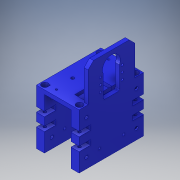
# Autodesk Inventor part: КВ33.044.501 - Каретка оси Y
Saved by Autodesk Inventor 2019 (Build 230136000, 136)
## iProperties
Created: 2019-07-21
Part Number: КВ33.044.501 - Каретка оси Y
Material: Пластик АБС
Document SubType Name: Modeling
Designer: Петров Иван
Density: 1.06 g/cm^3
Appearance: Синий — малярная краска — глянцевая
Mass: 139.056 g
Surface Area: 506.094 cm^2
Volume: 131.185 cm^3
Author: Петров Иван
Autodesk Inventor part; units mm, degrees
(part 1 of 2)
ref_plane "YZ Plane" through (0, 0, 0) normal (1, 0, 0) x (0, 1, 0)
ref_plane "XZ Plane" through (0, 0, 0) normal (0, 1, 0) x (-1, 0, 0)
ref_plane "XY Plane" through (0, 0, 0) normal (0, 0, 1) x (1, 0, 0)
sketch "Эскиз1" plane through (0, 0, 0) normal (1, 0, 0) x (0, 1, 0)
  line L0 (-34, 40) -> (34, 40)
  line L1 (34, 40) -> (34, -40)
  line L2 (34, -40) -> (-34, -40)
  line L3 (-34, -40) -> (-34, 40)
  line L4 (-34, 40) -> (34, -40) construction
  line L5 (34, 40) -> (-34, -40) construction
  line L6 (0, 0) -> (0, 31)
  line L7 (0, 31) -> (21.3, 31)
  line L8 (0, 31) -> (-21.3, 31)
  line L9 (0, 0) -> (0, -31)
  line L10 (0, -31) -> (21.3, -31)
  line L11 (0, -31) -> (-21.3, -31)
  circle A0 centre (21.3, 31) radius 2.1
  circle A1 centre (-21.3, 31) radius 2.1
  circle A2 centre (21.3, -31) radius 2.1
  circle A3 centre (-21.3, -31) radius 2.1
  dimension "d0" = 68
  dimension "d1" = 80
  dimension "d2" = 21.3
  dimension "d3" = 21.3
  dimension "d4" = 31
  dimension "d5" = 31
  dimension "d6" = 21.3
  dimension "d7" = 21.3
  dimension "d8" = 4.2
  dimension "d9" = 4.2
  dimension "d10" = 4.2
  dimension "d11" = 4.2
  constraints: 24 end point, 4 centre point, 4 coincident, 3 horizontal, 3 perpendicular, 2 midpoint, 2 parallel, 2 vertical
  measures "d0" distance of L1.end L2.end
  measures "d1" distance of L0.end L1.end
  measures "d2" distance of L6.end L7.end
  measures "d3" distance of L6.end L8.end
  measures "d4" distance of L6.start L6.end
  measures "d5" distance of L6.start L9.end
  measures "d6" distance of L9.end L10.end
  measures "d7" distance of L9.end L11.end
  measures "d8" diameter of A0
  measures "d9" diameter of A1
  measures "d10" diameter of A2
  measures "d11" diameter of A3
extrude "Выдавливание1" add sketch "Эскиз1" along normal blind 10
sketch "Эскиз2" plane through (10, 0, 0) normal (1, 0, 0) x (0, 0, -1)
  line L0 (-40, 34) -> (-40, -34) projected
  line L1 (-40, 0) -> (-40, 5)
  line L2 (-40, 0) -> (-26, 0)
  line L3 (-26, 0) -> (-26, 11)
  line L4 (-40, 5) -> (-26, 5)
  line L5 (-26, 5) -> (-26, 11)
  line L6 (-26, 11) -> (-40, 11)
  line L7 (-40, 11) -> (-40, 5)
  line L8 (-40, 0) -> (-40, -5)
  line L9 (-26, 0) -> (-26, -11)
  line L10 (-40, -5) -> (-26, -5)
  line L11 (-26, -5) -> (-26, -11)
  line L12 (-26, -11) -> (-40, -11)
  line L13 (-40, -11) -> (-40, -5)
  line L14 (40, -34) -> (40, 34) projected
  line L15 (40, 0) -> (40, 5)
  line L16 (40, 0) -> (26, 0)
  line L17 (26, 0) -> (26, 11)
  line L18 (26, 11) -> (40, 11)
  line L19 (40, 11) -> (40, 5)
  line L20 (40, 5) -> (26, 5)
  line L21 (26, 5) -> (26, 11)
  line L22 (26, 0) -> (26, -11)
  line L23 (40, 0) -> (40, -5)
  line L24 (26, -11) -> (40, -11)
  line L25 (40, -11) -> (40, -5)
  line L26 (40, -5) -> (26, -5)
  line L27 (26, -5) -> (26, -11)
  point P0 (0, 0)
  dimension "d14" = 5
  dimension "d15" = 14
  dimension "d16" = 11
  dimension "d17" = 5
  dimension "d18" = 11
  dimension "d19" = 5
  dimension "d20" = 14
  dimension "d21" = 11
  dimension "d22" = 11
  dimension "d23" = 5
  constraints: 52 end point, 8 parallel, 7 perpendicular, 5 horizontal, 4 point on line, 2 midpoint, 2 vertical
  measures "d14" distance of L1.start L1.end
  measures "d15" distance of L1.start L2.end
  measures "d16" distance of L2.end L3.end
  measures "d17" distance of L1.start L8.end
  measures "d18" distance of L2.end L9.end
  measures "d19" distance of L15.start L15.end
  measures "d20" distance of L15.start L16.end
  measures "d21" distance of L16.end L17.end
  measures "d22" distance of L16.end L22.end
  measures "d23" distance of L15.start L23.end
extrude "Выдавливание2" cut sketch "Эскиз2" against normal blind 10 contours L6 L3 L4 L0 | L10 L9 L12 L0 | L24 L22 L26 L14 | L20 L17 L18 L14
sketch "Эскиз3" plane through (0, 34, 40) normal (0, 1, 0) x (1, 0, 0)
  line L0 (0, 0) -> (10, 0) projected
  line L1 (5, 0) -> (5, 11.1)
  line L2 (0, 11.1) -> (10, 11.1) projected
  circle A0 centre (5, 5.55) radius 1.8
  line L3 (0, 80) -> (10, 80) projected
  line L4 (5, 80) -> (5, 68.9)
  line L5 (0, 68.9) -> (10, 68.9) projected
  circle A1 centre (5, 74.45) radius 1.8
  point P0 (0, 40)
  dimension "d26" = 3.6
  dimension "d29" = 3.6
  constraints: 6 midpoint, 4 end point, 2 centre point
  measures "d26" diameter of A0
  measures "d29" diameter of A1
extrude "Выдавливание3" cut sketch "Эскиз3" against normal through all
sketch "Эскиз4" plane through (0, 34, 40) normal (0, 1, 0) x (1, 0, 0)
  circle A0 centre (5, 5.55) radius 1.8 projected
  circle A1 centre (5, 5.55) radius 4
  circle A2 centre (5, 74.45) radius 1.8 projected
  circle A3 centre (5, 74.45) radius 4
  point P0 (0, 40)
  dimension "d30" = 8
  dimension "d31" = 8
  constraints: 2 centre point, 2 coincident
  measures "d30" diameter of A1
  measures "d31" diameter of A3
extrude "Выдавливание4" cut sketch "Эскиз4" against normal blind 10
sketch "Эскиз5" plane through (10, 0, 0) normal (1, 0, 0) x (0, 0, -1)
  line L0 (0, 0) -> (0, 18)
  line L1 (0, 18) -> (0, 20)
  line L2 (0, 20) -> (-15, 20)
  line L3 (-15, 20) -> (15, 20)
  circle A0 centre (-15, 20) radius 1.5
  circle A1 centre (15, 20) radius 1.5
  line L4 (0, 0) -> (6.6954, 0)
  line L5 (0, -18) -> (0, -20)
  line L6 (0, -20) -> (-15, -20)
  line L7 (-15, -20) -> (15, -20)
  circle A2 centre (-15, -20) radius 1.5
  circle A3 centre (15, -20) radius 1.5
  dimension "d34" = 18
  dimension "d35" = 2
  dimension "d36" = 15
  dimension "d37" = 30
  dimension "d38" = 3
  dimension "d39" = 3
  constraints: 16 end point, 6 symmetric about line, 4 centre point, 4 coincident, 3 point on line, 2 horizontal, 1 vertical, 2 other
  measures "d34" distance of L0.start L0.end
  measures "d35" distance of L0.end L1.end
  measures "d36" distance of L1.end L2.end
  measures "d37" distance of L2.end L3.end
  measures "d38" diameter of A0
  measures "d39" diameter of A1
extrude "Выдавливание5" cut sketch "Эскиз5" against normal blind 10 contours A2 | A3
sketch "Эскиз6" plane through (10, 0, 0) normal (1, 0, 0) x (0, 0, -1)
  circle A0 centre (15, -20) radius 1.5 projected
  circle A1 centre (-15, -20) radius 1.5 projected
  circle A2 centre (-31, 21.3) radius 2.1 projected
  circle A3 centre (-31, -21.3) radius 2.1 projected
  circle A4 centre (31, 21.3) radius 2.1 projected
  circle A5 centre (31, -21.3) radius 2.1 projected
  line L0 (-40, 11) -> (-26, 11) projected
  line L1 (-26, 11) -> (-26, 5) projected
  line L2 (-26, 5) -> (-40, 5) projected
  line L3 (-40, 5) -> (-40, -5) projected
  line L4 (-40, -5) -> (-26, -5) projected
  line L5 (-26, -5) -> (-26, -11) projected
  line L6 (-26, -11) -> (-40, -11) projected
  line L7 (-40, -11) -> (-40, -34) projected
  line L8 (-40, -34) -> (40, -34) projected
  line L9 (40, -34) -> (40, -11) projected
  line L10 (40, -11) -> (26, -11) projected
  line L11 (26, -11) -> (26, -5) projected
  line L12 (26, -5) -> (40, -5) projected
  line L13 (40, -5) -> (40, 5) projected
  line L14 (40, 5) -> (26, 5) projected
  line L15 (26, 5) -> (26, 11) projected
  line L16 (26, 11) -> (40, 11) projected
  line L17 (40, 11) -> (40, 34) projected
  line L18 (40, 34) -> (-40, 34) projected
  line L19 (-40, 34) -> (-40, 11) projected
  point P0 (0, 0)
sketch "Эскиз8" plane through (0, 0, 0) normal (-1, 0, 0) x (0, 0, 1)
  line L0 (-40, 34) -> (-40, 11) projected
  line L1 (40, 11) -> (40, 34) projected
  line L2 (-40, 34) -> (40, 34)
  line L3 (40, 34) -> (40, 29)
  line L4 (40, 29) -> (-40, 29)
  line L5 (-40, 29) -> (-40, 34)
  point P0 (0, 0)
  dimension "d46" = 5
  constraints: 8 end point, 2 parallel, 1 horizontal, 1 perpendicular, 1 point on line
  measures "d46" distance of L2.end L3.end
extrude "Выдавливание7" add sketch "Эскиз8" along normal blind 33
sketch "Эскиз13" plane through (-33, 0, 0) normal (-1, 0, 0) x (0, 0, 1)
  circle A0 centre (15, -20) radius 1.5
  circle A1 centre (-15, -20) radius 1.5
  circle A2 centre (-31, 21.3) radius 2.1
  circle A3 centre (-31, -21.3) radius 2.1
  circle A4 centre (31, 21.3) radius 2.1
  circle A5 centre (31, -21.3) radius 2.1
  line L0 (-40, 11) -> (-26, 11)
  line L1 (-26, 11) -> (-26, 5)
  line L2 (-26, 5) -> (-40, 5)
  line L3 (-40, 5) -> (-40, -5)
  line L4 (-40, -5) -> (-26, -5)
  line L5 (-26, -5) -> (-26, -11)
  line L6 (-26, -11) -> (-40, -11)
  line L7 (-40, -11) -> (-40, -34)
  line L8 (-40, -34) -> (40, -34)
  line L9 (40, -34) -> (40, -11)
  line L10 (40, -11) -> (26, -11)
  line L11 (26, -11) -> (26, -5)
  line L12 (26, -5) -> (40, -5)
  line L13 (40, -5) -> (40, 5)
  line L14 (40, 5) -> (26, 5)
  line L15 (26, 5) -> (26, 11)
  line L16 (26, 11) -> (40, 11)
  line L17 (40, 11) -> (40, 34)
  line L18 (40, 34) -> (-40, 34)
  line L19 (-40, 34) -> (-40, 11)
  point P0 (0, 0)
  point P1 (0, 0)
  constraints: 40 end point, 6 centre point
extrude "Выдавливание11" add sketch "Эскиз13" along normal blind 10
sketch "Эскиз14" plane through (10, 34, 40) normal (0, 1, 0) x (1, 0, 0)
  line L0 (0, 80) -> (-53, 80) projected
  line L1 (-26.5, 80) -> (-26.5, 69.4857)
  circle A0 centre (-5, 5.55) radius 4 projected
  circle A1 centre (-5, 74.45) radius 4 projected
  line L2 (0, 0) -> (-53, 0) projected
  line L3 (0, 80) -> (0, 0) projected
  line L4 (0, 80) -> (-53, 80) projected
  line L5 (-53, 0) -> (-53, 80) projected
  circle A2 centre (-5, 5.55) radius 1.8 projected
  circle A3 centre (-5, 74.45) radius 1.8 projected
  circle A4 centre (-48, 5.55) radius 1.8
  circle A5 centre (-48, 74.45) radius 1.8
  point P0 (-10, 40)
  constraints: 2 centre point, 2 end point, 2 symmetric about line, 1 midpoint, 1 vertical, 2 other
extrude "Выдавливание12" cut sketch "Эскиз14" against normal through all contours A4 | A5
sketch "Эскиз15" plane through (10, 34, 40) normal (0, 1, 0) x (1, 0, 0)
  circle A0 centre (-48, 74.45) radius 1.8 projected
  circle A1 centre (-48, 74.45) radius 4
  circle A2 centre (-48, 5.55) radius 1.8 projected
  circle A3 centre (-48, 5.55) radius 4
  point P0 (-10, 40)
  dimension "d65" = 8
  dimension "d66" = 8
  constraints: 2 centre point, 2 coincident
  measures "d65" diameter of A1
  measures "d66" diameter of A3
extrude "Выдавливание13" cut sketch "Эскиз15" against normal blind 20
sketch "Эскиз16" plane through (10, 34, 40) normal (0, 1, 0) x (1, 0, 0)
  circle A0 centre (-48, 74.45) radius 4 projected
  circle A1 centre (-48, 5.55) radius 4 projected
  circle A2 centre (-5, 5.55) radius 4 projected
  circle A3 centre (-5, 74.45) radius 4 projected
  line L0 (0, 0) -> (-53, 0) projected
  line L1 (0, 80) -> (0, 0) projected
  line L2 (0, 80) -> (-53, 80) projected
  line L3 (-53, 0) -> (-53, 80) projected
  point P0 (-10, 40)
sketch "Эскиз17" plane through (-33, -34, -40) normal (0, -1, 0) x (1, 0, 0)
  circle A0 centre (-5, 5.55) radius 4
  circle A1 centre (-5, 74.45) radius 4
  circle A2 centre (-5, 5.55) radius 1.8 projected
  line L0 (-5, 5.55) -> (-5, 18.1127)
  circle A3 centre (38, 74.45) radius 4
  circle A4 centre (38, 5.55) radius 4
  circle A5 centre (-5, 5.55) radius 4
  circle A6 centre (-5, 74.45) radius 4
  line L1 (-10, 0) -> (43, 0)
  line L2 (-10, 80) -> (-10, 0)
  line L3 (-10, 80) -> (43, 80)
  line L4 (43, 0) -> (43, 80)
  circle A7 centre (-5, 5.55) radius 1.8
  point P0 (33, 40)
  point P1 (-10, 40)
  point P2 (0, 40)
  constraints: 10 end point, 7 centre point, 1 symmetric about line, 1 vertical, 3 other
extrude "Выдавливание14" cut sketch "Эскиз17" against normal blind 20 contours A0 | A1 | A3 | A4
sketch "Эскиз25" plane through (10, 34, 40) normal (0, 1, 0) x (1, 0, 0)
  line L0 (-10, 68.9) -> (0, 68.9) projected
  line L1 (-10, 11.1) -> (0, 11.1) projected
  line L2 (-5, 68.9) -> (0, 68.9)
  line L3 (0, 68.9) -> (0, 11.1)
  line L4 (0, 11.1) -> (-5, 11.1)
  line L5 (-5, 11.1) -> (-5, 68.9)
  point P0 (-10, 40)
  constraints: 8 end point, 2 parallel, 1 horizontal, 1 midpoint, 1 perpendicular, 1 point on line
extrude "Выдавливание21" add sketch "Эскиз25" along normal blind 40
sketch "Эскиз26" plane through (10, 0, 0) normal (1, 0, 0) x (0, 0, -1)
  line L0 (-12.6, 44.2) -> (-14.9, 44.2)
  line L1 (-12.6, 44.2) -> (-12.6, 42.8)
  line L2 (-14.9, 42.8) -> (-12.6, 42.8)
  line L3 (-14.9, 36.2) -> (-14.9, 42.8)
  line L4 (-12.6, 36.2) -> (-14.9, 36.2)
  circle A0 centre (0, 62) radius 9.15
  circle A1 centre (0, 62) radius 1.5
  circle A2 centre (8, 26) radius 1.3
  circle A3 centre (13.5, 39.5) radius 1.3
  circle A4 centre (13.5, 31.5) radius 1.3
  circle A5 centre (13.5, 47.5) radius 1.3
  circle A6 centre (13.5, 55.5) radius 1.3
  circle A7 centre (-8, 26) radius 1.3
  circle A8 centre (-13.5, 39.5) radius 1.3
  circle A9 centre (-13.5, 31.5) radius 1.3
  circle A10 centre (-13.5, 47.5) radius 1.3
  circle A11 centre (-13.5, 55.5) radius 1.3
  line L5 (-0.1, 73.0198) -> (-0.1, 72.4796)
  line L6 (-7, 73.0198) -> (-0.1, 73.0198)
  arc A12 (-7, 73.0198) -> (-7.75, 72.9686) centre (-7, 67.5) ccw
  line L7 (-7.75, 70.5) -> (-7.75, 72.9686)
  arc A13 (-9.5, 68.75) -> (-7.75, 70.5) centre (-9.5, 70.5) ccw
  line L8 (-10, 68.75) -> (-9.5, 68.75)
  line L9 (-10, 31.1937) -> (-10, 68.75)
  arc A14 (-10, 31.1937) -> (-9.6078, 30.5055) centre (-9.2, 31.1937) ccw
  arc A15 (-9.6078, 30.5055) -> (-8.9945, 29.8922) centre (-10.5, 29) ccw
  arc A16 (-8.9945, 29.8922) -> (-8.3063, 29.5) centre (-8.3063, 30.3) ccw
  line L10 (8.3063, 29.5) -> (-8.3063, 29.5)
  arc A17 (8.3063, 29.5) -> (8.9945, 29.8922) centre (8.3063, 30.3) ccw
  arc A18 (9.6078, 30.5055) -> (8.9945, 29.8922) centre (10.5, 29) ccw
  arc A19 (8.9945, 29.8922) -> (9.6078, 30.5055) centre (10.5, 29) ccw
  line L11 (-11.3229, 68.75) -> (-10, 68.75)
  arc A20 (-11.3229, 68.75) -> (-11.5, 67.4989) centre (-6.9922, 67.4989) ccw
  line L12 (-11.5, 67.4989) -> (-11.5, 60)
  line L13 (-12.6, 60) -> (-11.5, 60)
  line L14 (-12.6, 58.8) -> (-12.6, 60)
  line L15 (-14.9, 58.8) -> (-12.6, 58.8)
  line L16 (-14.9, 52.2) -> (-14.9, 58.8)
  line L17 (-12.6, 52.2) -> (-14.9, 52.2)
  line L18 (-12.6, 50.8) -> (-12.6, 52.2)
  line L19 (-14.9, 50.8) -> (-12.6, 50.8)
  line L20 (-14.9, 44.2) -> (-14.9, 50.8)
  line L21 (-12.6, 44.2) -> (-14.9, 44.2)
  line L22 (-12.6, 42.8) -> (-12.6, 44.2)
  line L23 (-14.9, 42.8) -> (-12.6, 42.8)
  line L24 (-14.9, 36.2) -> (-14.9, 42.8)
  line L25 (-12.6, 36.2) -> (-14.9, 36.2)
  line L26 (-12.6, 34.8) -> (-12.6, 36.2)
  line L27 (-14.9, 34.8) -> (-12.6, 34.8)
  line L28 (-14.9, 28.2) -> (-14.9, 34.8)
  line L29 (-12.6, 28.2) -> (-14.9, 28.2)
  line L30 (-12.6, 26.9802) -> (-12.6, 28.2)
  arc A21 (-12.6, 26.9802) -> (-12.5198, 26.9) centre (-11.5, 28) ccw
  line L31 (-11.3, 26.9) -> (-12.5198, 26.9)
  line L32 (-11.3, 24.6) -> (-11.3, 26.9)
  line L33 (-4.7, 24.6) -> (-11.3, 24.6)
  line L34 (-4.7, 26.9) -> (-4.7, 24.6)
  line L35 (4.7, 26.9) -> (-4.7, 26.9)
  line L36 (4.7, 24.6) -> (4.7, 26.9)
  line L37 (11.3, 24.6) -> (4.7, 24.6)
  line L38 (11.3, 26.9) -> (11.3, 24.6)
  line L39 (12.5198, 26.9) -> (11.3, 26.9)
  arc A22 (12.5198, 26.9) -> (12.6, 26.9802) centre (11.5, 28) ccw
  line L40 (12.6, 28.2) -> (12.6, 26.9802)
  line L41 (14.9, 28.2) -> (12.6, 28.2)
  line L42 (14.9, 34.8) -> (14.9, 28.2)
  line L43 (12.6, 34.8) -> (14.9, 34.8)
  line L44 (12.6, 36.2) -> (12.6, 34.8)
  line L45 (14.9, 36.2) -> (12.6, 36.2)
  line L46 (14.9, 42.8) -> (14.9, 36.2)
  line L47 (12.6, 42.8) -> (14.9, 42.8)
  line L48 (12.6, 44.2) -> (12.6, 42.8)
  line L49 (14.9, 44.2) -> (12.6, 44.2)
  line L50 (14.9, 50.8) -> (14.9, 44.2)
  line L51 (12.6, 50.8) -> (14.9, 50.8)
  line L52 (12.6, 52.2) -> (12.6, 50.8)
  line L53 (14.9, 52.2) -> (12.6, 52.2)
  line L54 (14.9, 58.8) -> (14.9, 52.2)
  line L55 (12.6, 58.8) -> (14.9, 58.8)
  line L56 (12.6, 60) -> (12.6, 58.8)
  line L57 (11.5, 60) -> (12.6, 60)
  line L58 (11.5, 67.5) -> (11.5, 60)
  arc A23 (11.5, 67.5) -> (11.3229, 68.75) centre (6.9922, 67.4989) ccw
  line L59 (10, 68.75) -> (11.3229, 68.75)
  line L60 (9.5, 68.75) -> (10, 68.75)
  arc A24 (7.75, 70.5) -> (9.5, 68.75) centre (9.5, 70.5) ccw
  line L61 (7.75, 72.9686) -> (7.75, 70.5)
  arc A25 (7.75, 72.9686) -> (7, 73.0198) centre (7, 67.5) ccw
  line L62 (0.1, 73.0198) -> (7, 73.0198)
  line L63 (0.1, 72.4796) -> (0.1, 73.0198)
  arc A26 (-8.9945, 29.8922) -> (-9.6078, 30.5055) centre (-10.5, 29) ccw
  arc A27 (9.6078, 30.5055) -> (10, 31.1895) centre (9.2, 31.1937) ccw
  line L64 (10, 68.75) -> (10, 31.1895)
  line L65 (0, 0) -> (0, 74)
  line L66 (28.9, 74) -> (-28.9, 74) projected
  line L67 (0, 74) -> (0, 62)
  line L68 (-9.15, 62) -> (-10, 62)
  line L69 (9.15, 62) -> (10, 62)
  point P0 (0, 62)
  dimension "d102" = 12
  constraints: 138 end point, 34 point on circle, 28 centre point, 5 point on line, 1 midpoint, 1 perpendicular
  measures "d102" distance of L65.end L67.end
extrude "Выдавливание22" cut sketch "Эскиз26" against normal blind 5 contours L68 A0 L65 L10 A16 A26 A14 L9 | A0 L65 A1 | A0 L65 A1 | A0 L69 L64 A27 A18 A17 L10 L65 | L65 A1 | A1 L65 | A3 | A5 | A6 | A8 | A10 | A11
sketch "Эскиз29" plane through (-43, 34, -40) normal (0, 1, 0) x (1, 0, 0)
  line L0 (43, -11.1) -> (53, -11.1) projected
  line L1 (48, -11.1) -> (48, -68.9) projected
  line L2 (48, -11.1) -> (48, -68.9)
  circle A0 centre (40.9968, -58.9777) radius 1.5
  line L3 (33.923, -34.3302) -> (33.923, -66.4777)
  line L4 (33.923, -66.4777) -> (47.9968, -66.4777)
  line L5 (47.9968, -66.4777) -> (47.9968, -34.3302)
  line L6 (47.9968, -34.3302) -> (33.923, -34.3302)
  point P0 (43, -40)
  point P1 (40.9968, -50.4777)
  constraints: 10 end point, 1 centre point, 1 collinear, 1 midpoint
extrude "Выдавливание23" cut sketch "Эскиз29" against normal blind 4 contours A0 | L6 L5 L4 L3
chamfer "Фаска5" distance 2.75 angle 45 2 edges at (7.5, 74, 28.9) (7.5, 74, -28.9)
sketch "Эскиз43" plane through (-43, 34, 40) normal (0, 1, 0) x (1, 0, 0)
  line L0 (1.9345, -0.1187) -> (2.4471, -0.1187)
  line L1 (2.4471, -0.1187) -> (2.5388, 1.3153)
  arc A0 (6.7302, 1.3153) -> (2.5388, 1.3153) centre (4.6345, 1.1813) ccw
  line L2 (6.7302, 1.3153) -> (6.8219, -0.1187)
  line L3 (6.8219, -0.1187) -> (11.1103, -0.1187)
  arc A1 (11.1103, -0.1187) -> (11.181, -0.0894) centre (11.1103, -0.0187) ccw
  line L4 (11.181, -0.0894) -> (11.5052, 0.2348)
  arc A2 (11.8588, 0.3813) -> (11.5052, 0.2348) centre (11.8588, -0.1187) ccw
  line L5 (11.8588, 0.3813) -> (21.5345, 0.3813)
  arc A3 (21.5345, 0.3813) -> (21.4407, 0.4466) centre (21.5345, 0.4813) ccw
  line L6 (21.4407, 0.4466) -> (21.4407, 9.5417)
  arc A4 (21.4407, 9.5417) -> (21.4519, 9.7313) centre (21.5345, 9.6313) ccw
  line L7 (21.4519, 9.7313) -> (18.6088, 9.7313)
  arc A5 (18.2552, 9.8777) -> (18.6088, 9.7313) centre (18.6088, 10.2313) ccw
  line L8 (18.2552, 9.8777) -> (17.931, 10.202)
  arc A6 (17.931, 10.202) -> (17.8603, 10.2313) centre (17.8603, 10.1313) ccw
  line L9 (17.8603, 10.2313) -> (15.1088, 10.2313)
  arc A7 (15.1088, 10.2313) -> (15.0381, 10.202) centre (15.1088, 10.1313) ccw
  line L10 (15.0381, 10.202) -> (14.7138, 9.8777)
  arc A8 (14.3603, 9.7313) -> (14.7138, 9.8777) centre (14.3603, 10.2313) ccw
  line L11 (14.3603, 9.7313) -> (9.1088, 9.7313)
  arc A9 (8.7552, 9.8777) -> (9.1088, 9.7313) centre (9.1088, 10.2313) ccw
  line L12 (8.7552, 9.8777) -> (8.431, 10.202)
  arc A10 (8.431, 10.202) -> (8.3603, 10.2313) centre (8.3603, 10.1313) ccw
  line L13 (8.3603, 10.2313) -> (5.6088, 10.2313)
  arc A11 (5.6088, 10.2313) -> (5.5381, 10.202) centre (5.6088, 10.1313) ccw
  line L14 (5.5381, 10.202) -> (5.2138, 9.8777)
  arc A12 (4.8603, 9.7313) -> (5.2138, 9.8777) centre (4.8603, 10.2313) ccw
  line L15 (4.8603, 9.7313) -> (1.9345, 9.7313)
  arc A13 (1.9345, 9.7313) -> (2.0046, 9.5599) centre (1.9345, 9.6313) ccw
  line L16 (2.0046, 9.5599) -> (2.0046, 0.0526)
  arc A14 (2.0046, 0.0526) -> (1.9345, -0.1187) centre (1.9345, -0.0187) ccw
  circle A15 centre (7.7854, 7.6813) radius 1.25
  circle A16 centre (17.2854, 7.6813) radius 1.25
  line L17 (18.4587, 5.4313) -> (17.8421, 4.1313)
  line L18 (17.8421, 4.1313) -> (17.8254, 4.1313)
  line L19 (17.8254, 4.1313) -> (17.2254, 5.4313)
  line L20 (17.2254, 5.4313) -> (17.3522, 5.4313)
  line L21 (17.3522, 5.4313) -> (17.5444, 5.0146)
  line L22 (17.5444, 5.0146) -> (18.1337, 5.0146)
  line L23 (18.1337, 5.0146) -> (18.3314, 5.4313)
  line L24 (18.3314, 5.4313) -> (18.4587, 5.4313)
  spline S0 degree 3 poles (15.6387, 4.4948) (15.639, 4.4859) (15.6394, 4.4685) (15.6435, 4.4428) (15.6497, 4.4181) (15.6586, 4.3942) (15.6704, 4.3714) (15.6847, 4.3496) (15.7012, 4.3285) (15.7202, 4.3088) (15.7412, 4.2907) (15.7633, 4.2747) (15.7867, 4.2613) (15.8113, 4.2503) (15.8371, 4.2417) (15.8639, 4.2358) (15.8919, 4.232) (15.911, 4.2315) (15.9208, 4.2313) knots 0 0 0 0 0.061965 0.122122 0.180988 0.239933 0.299906 0.359989 0.421776 0.486576 0.551535 0.615018 0.677259 0.73973 0.80305 0.866495 0.931973 1 1 1 1
  spline S1 degree 3 poles (15.9208, 4.2313) (15.9309, 4.2315) (15.9509, 4.2321) (15.9802, 4.2357) (16.0082, 4.242) (16.0349, 4.2506) (16.0603, 4.2615) (16.0844, 4.2752) (16.1071, 4.2914) (16.1284, 4.3099) (16.148, 4.3304) (16.1653, 4.3533) (16.1803, 4.3781) (16.1935, 4.4048) (16.2042, 4.4336) (16.2123, 4.4644) (16.2188, 4.4971) (16.221, 4.5197) (16.2221, 4.5313) knots 0 0 0 0 0.064439 0.126547 0.186887 0.245878 0.304041 0.362191 0.420976 0.48066 0.5406 0.600689 0.661936 0.724443 0.789038 0.856314 0.926352 1 1 1 1
  line L25 (16.2221, 4.5313) -> (16.3387, 4.5313)
  spline S2 degree 3 poles (16.3387, 4.5313) (16.338, 4.5158) (16.3365, 4.4854) (16.3295, 4.4411) (16.3195, 4.3987) (16.3053, 4.3586) (16.2878, 4.3205) (16.2667, 4.2845) (16.2417, 4.2507) (16.2134, 4.2194) (16.1827, 4.1908) (16.1495, 4.166) (16.1147, 4.1451) (16.0782, 4.1276) (16.0398, 4.1145) (15.9997, 4.1047) (15.9578, 4.0989) (15.9293, 4.0983) (15.9148, 4.0979) knots 0 0 0 0 0.068791 0.135103 0.198979 0.261904 0.323495 0.385195 0.446969 0.509765 0.572251 0.633405 0.693251 0.752583 0.812579 0.873275 0.93555 1 1 1 1
  spline S3 degree 3 poles (15.9148, 4.0979) (15.9005, 4.0983) (15.8725, 4.0989) (15.8316, 4.1046) (15.7927, 4.1134) (15.7558, 4.1257) (15.7213, 4.1424) (15.6888, 4.1624) (15.658, 4.1855) (15.6303, 4.2127) (15.6049, 4.2417) (15.5829, 4.2727) (15.5641, 4.3048) (15.5485, 4.3381) (15.5369, 4.3729) (15.5282, 4.4089) (15.5232, 4.4462) (15.5224, 4.4715) (15.5221, 4.4844) knots 0 0 0 0 0.069475 0.136517 0.200789 0.26383 0.325735 0.387291 0.449509 0.512968 0.576275 0.63758 0.697903 0.757172 0.816599 0.876653 0.93729 1 1 1 1
  spline S4 degree 3 poles (15.5221, 4.4844) (15.5227, 4.5025) (15.5239, 4.5384) (15.5346, 4.5911) (15.5513, 4.6422) (15.5713, 4.6834) (15.5915, 4.7165) (15.6098, 4.7438) (15.6311, 4.7732) (15.6559, 4.8046) (15.6836, 4.8382) (15.7144, 4.874) (15.7486, 4.9117) (15.7726, 4.9375) (15.7851, 4.9508) knots 0 0 0 0 0.098702 0.195672 0.292422 0.391343 0.444462 0.504229 0.570352 0.642546 0.722288 0.807921 0.90047 1 1 1 1
  line L26 (15.7851, 4.9508) -> (16.1103, 5.2979)
  line L27 (16.1103, 5.2979) -> (15.5054, 5.2979)
  line L28 (15.5054, 5.2979) -> (15.5054, 5.4313)
  line L29 (15.5054, 5.4313) -> (16.3887, 5.4313)
  line L30 (16.3887, 5.4313) -> (15.8846, 4.8932)
  spline S5 degree 3 poles (15.8846, 4.8932) (15.8723, 4.8804) (15.8487, 4.8558) (15.8154, 4.8199) (15.7854, 4.7866) (15.7587, 4.7559) (15.7357, 4.7274) (15.7153, 4.7021) (15.699, 4.6788) (15.6813, 4.6518) (15.6641, 4.6188) (15.6493, 4.5785) (15.6404, 4.537) (15.6393, 4.5089) (15.6387, 4.4948) knots 0 0 0 0 0.110803 0.212829 0.306101 0.390647 0.466924 0.534481 0.593587 0.644557 0.7362 0.825024 0.911986 1 1 1 1
  line L31 (15.1287, 4.7813) -> (14.9954, 4.1313)
  line L32 (14.9954, 4.1313) -> (14.4621, 4.1313)
  line L33 (14.4621, 4.1313) -> (14.4621, 4.2646)
  line L34 (14.4621, 4.2646) -> (14.9042, 4.2646)
  line L35 (14.9042, 4.2646) -> (14.9743, 4.6065)
  spline S6 degree 3 poles (14.9743, 4.6065) (14.9605, 4.6027) (14.9339, 4.5954) (14.8945, 4.5872) (14.8572, 4.5823) (14.8329, 4.5816) (14.8212, 4.5813) knots 0 0 0 0 0.275068 0.532901 0.773973 1 1 1 1
  spline S7 degree 3 poles (14.8212, 4.5813) (14.8067, 4.5816) (14.7781, 4.5822) (14.7364, 4.5881) (14.6965, 4.5975) (14.6586, 4.6105) (14.6226, 4.6272) (14.5889, 4.648) (14.5569, 4.6724) (14.5272, 4.7004) (14.5003, 4.7312) (14.4766, 4.7643) (14.4565, 4.7994) (14.4403, 4.8368) (14.4274, 4.8762) (14.4188, 4.9179) (14.413, 4.9615) (14.4124, 4.9913) (14.4121, 5.0065) knots 0 0 0 0 0.065808 0.129394 0.190894 0.251281 0.310815 0.370371 0.430768 0.492881 0.555104 0.616067 0.677256 0.73826 0.800762 0.864778 0.931045 1 1 1 1
  spline S8 degree 3 poles (14.4121, 5.0065) (14.4123, 5.0171) (14.4128, 5.0382) (14.4153, 5.0694) (14.4201, 5.1) (14.4266, 5.1299) (14.4349, 5.1592) (14.4451, 5.1878) (14.4575, 5.2155) (14.4711, 5.2428) (14.4864, 5.2688) (14.5034, 5.2932) (14.5214, 5.3163) (14.5407, 5.3378) (14.5616, 5.3576) (14.5837, 5.3757) (14.607, 5.3926) (14.6318, 5.4075) (14.6574, 5.4213) (14.6844, 5.4325) (14.7121, 5.4426) (14.7408, 5.4506) (14.7706, 5.4569) (14.8014, 5.4612) (14.8331, 5.4643) (14.8546, 5.4645) (14.8654, 5.4646) knots 0 0 0 0 0.044014 0.087434 0.130118 0.172554 0.214555 0.256298 0.298438 0.340849 0.382715 0.423924 0.464246 0.504074 0.543862 0.583567 0.623094 0.663229 0.703551 0.743938 0.784541 0.82575 0.867757 0.910745 0.954914 1 1 1 1
  spline S9 degree 3 poles (14.8654, 5.4646) (14.8784, 5.4643) (14.9039, 5.4638) (14.9412, 5.4586) (14.9771, 5.451) (15.0114, 5.4396) (15.0442, 5.4254) (15.0752, 5.4073) (15.1051, 5.3869) (15.1328, 5.3628) (15.1585, 5.3365) (15.1815, 5.3079) (15.2019, 5.2775) (15.2196, 5.2453) (15.2346, 5.2111) (15.2464, 5.1751) (15.256, 5.1372) (15.26, 5.1112) (15.2621, 5.0979) knots 0 0 0 0 0.065421 0.128708 0.190236 0.250724 0.310637 0.370766 0.431615 0.493523 0.555883 0.617342 0.678668 0.740711 0.802985 0.866803 0.932347 1 1 1 1
  line L36 (15.2621, 5.0979) -> (15.1454, 5.0979)
  spline S10 degree 3 poles (15.1454, 5.0979) (15.1425, 5.1103) (15.137, 5.1342) (15.1249, 5.1676) (15.1101, 5.1975) (15.0925, 5.2241) (15.0715, 5.2472) (15.0475, 5.2679) (15.0206, 5.2865) (14.9908, 5.3021) (14.9593, 5.3153) (14.9263, 5.3241) (14.8928, 5.3303) (14.8701, 5.331) (14.8587, 5.3313) knots 0 0 0 0 0.094687 0.181994 0.264377 0.34218 0.418618 0.496509 0.577369 0.661511 0.746733 0.831258 0.915206 1 1 1 1
  spline S11 degree 3 poles (14.8587, 5.3313) (14.8475, 5.331) (14.8256, 5.3304) (14.7934, 5.3257) (14.7623, 5.3186) (14.7326, 5.308) (14.7037, 5.295) (14.6766, 5.2784) (14.6502, 5.2593) (14.6256, 5.2374) (14.603, 5.2133) (14.583, 5.1875) (14.5664, 5.1599) (14.5523, 5.1312) (14.5417, 5.1008) (14.5341, 5.0691) (14.5297, 5.0358) (14.529, 5.0131) (14.5287, 5.0016) knots 0 0 0 0 0.064207 0.126425 0.18768 0.248216 0.308305 0.369661 0.431699 0.495947 0.559758 0.622295 0.683911 0.745092 0.80674 0.869087 0.93329 1 1 1 1
  spline S12 degree 3 poles (14.5287, 5.0016) (14.529, 4.9912) (14.5295, 4.9707) (14.5334, 4.9409) (14.5402, 4.9126) (14.5496, 4.8858) (14.5616, 4.8605) (14.5763, 4.8366) (14.5938, 4.8144) (14.6139, 4.7939) (14.6359, 4.775) (14.6602, 4.7589) (14.6863, 4.7454) (14.7139, 4.7337) (14.7436, 4.7253) (14.7749, 4.719) (14.808, 4.7154) (14.8306, 4.7149) (14.8423, 4.7146) knots 0 0 0 0 0.065351 0.127916 0.18836 0.247216 0.30563 0.36377 0.422661 0.482687 0.5433 0.604118 0.664965 0.727413 0.791468 0.858055 0.927037 1 1 1 1
  spline S13 degree 3 poles (14.8423, 4.7146) (14.8523, 4.7148) (14.8732, 4.7153) (14.9051, 4.7185) (14.9386, 4.7238) (14.9736, 4.7311) (15.0103, 4.7406) (15.0484, 4.752) (15.0882, 4.7657) (15.115, 4.776) (15.1287, 4.7813) knots 0 0 0 0 0.102203 0.211023 0.3251 0.446502 0.573788 0.708901 0.850358 1 1 1 1
  line L37 (11.6821, 5.4313) -> (11.0654, 4.1313)
  line L38 (11.0654, 4.1313) -> (11.0487, 4.1313)
  line L39 (11.0487, 4.1313) -> (10.4487, 5.4313)
  line L40 (10.4487, 5.4313) -> (10.5756, 5.4313)
  line L41 (10.5756, 5.4313) -> (10.7677, 5.0146)
  line L42 (10.7677, 5.0146) -> (11.3571, 5.0146)
  line L43 (11.3571, 5.0146) -> (11.5547, 5.4313)
  line L44 (11.5547, 5.4313) -> (11.6821, 5.4313)
  spline S14 degree 3 poles (10.1721, 4.7737) (10.1715, 4.7503) (10.1703, 4.7043) (10.1607, 4.6368) (10.1452, 4.5721) (10.1231, 4.5104) (10.0951, 4.4513) (10.0606, 4.3953) (10.0198, 4.342) (9.9732, 4.2922) (9.9221, 4.2467) (9.8674, 4.2066) (9.8092, 4.1733) (9.7481, 4.1454) (9.6837, 4.124) (9.616, 4.109) (9.5453, 4.0997) (9.4971, 4.0985) (9.4726, 4.0979) knots 0 0 0 0 0.064558 0.127014 0.187955 0.248014 0.307748 0.368235 0.42947 0.492743 0.556258 0.618217 0.679655 0.741246 0.803415 0.866815 0.932328 1 1 1 1
  spline S15 degree 3 poles (9.4726, 4.0979) (9.4576, 4.0981) (9.4281, 4.0985) (9.3843, 4.1019) (9.3418, 4.1077) (9.3003, 4.1155) (9.2598, 4.1253) (9.2205, 4.1379) (9.1822, 4.1524) (9.1451, 4.1691) (9.1095, 4.1879) (9.0753, 4.2085) (9.0428, 4.2309) (9.0118, 4.2549) (8.9828, 4.281) (8.955, 4.3086) (8.9292, 4.3384) (8.9134, 4.3593) (8.9054, 4.3698) knots 0 0 0 0 0.068548 0.135683 0.201215 0.265682 0.329267 0.392395 0.45507 0.517127 0.57879 0.63974 0.700192 0.759806 0.819628 0.879355 0.939512 1 1 1 1
  line L45 (8.9054, 4.3698) -> (9.0075, 4.4479)
  spline S16 degree 3 poles (9.0075, 4.4479) (9.0148, 4.4393) (9.0292, 4.422) (9.0525, 4.3978) (9.0768, 4.3751) (9.102, 4.3539) (9.1286, 4.3348) (9.1561, 4.3168) (9.1847, 4.3008) (9.2244, 4.2813) (9.2763, 4.2609) (9.3416, 4.2439) (9.4097, 4.233) (9.4562, 4.2319) (9.4799, 4.2313) knots 0 0 0 0 0.063163 0.125475 0.187121 0.248294 0.309295 0.36985 0.430973 0.492456 0.616148 0.740844 0.868183 1 1 1 1
  spline S17 degree 3 poles (9.4799, 4.2313) (9.4929, 4.2314) (9.5188, 4.2317) (9.5573, 4.2357) (9.5951, 4.2412) (9.6322, 4.2494) (9.6684, 4.2598) (9.7041, 4.2722) (9.7387, 4.2876) (9.7727, 4.3046) (9.8054, 4.3237) (9.8362, 4.3446) (9.8652, 4.3671) (9.8923, 4.3911) (9.9176, 4.4166) (9.941, 4.4438) (9.9622, 4.4727) (9.9818, 4.5029) (9.9993, 4.5343) (10.014, 4.5671) (10.027, 4.6005) (10.0373, 4.6351) (10.0454, 4.6706) (10.0511, 4.7071) (10.0549, 4.7445) (10.0552, 4.7698) (10.0554, 4.7826) knots 0 0 0 0 0.043955 0.087502 0.130463 0.172752 0.215403 0.25765 0.300153 0.343121 0.385925 0.427686 0.468818 0.509492 0.549883 0.58998 0.630405 0.670869 0.711384 0.751627 0.791776 0.832459 0.873319 0.914543 0.956924 1 1 1 1
  spline S18 degree 3 poles (10.0554, 4.7826) (10.0549, 4.8018) (10.054, 4.8395) (10.0458, 4.8948) (10.0334, 4.9477) (10.0147, 4.998) (9.9917, 5.0462) (9.9627, 5.0916) (9.929, 5.1349) (9.8903, 5.1749) (9.8478, 5.2115) (9.8022, 5.2437) (9.7536, 5.2706) (9.7026, 5.293) (9.6487, 5.3101) (9.5921, 5.3222) (9.5329, 5.3301) (9.4924, 5.3309) (9.4718, 5.3313) knots 0 0 0 0 0.064323 0.12629 0.186726 0.246146 0.305576 0.365429 0.426326 0.48884 0.551725 0.613919 0.675484 0.737334 0.800229 0.864502 0.931041 1 1 1 1
  spline S19 degree 3 poles (9.4718, 5.3313) (9.4491, 5.3306) (9.4044, 5.3294) (9.3389, 5.3189) (9.2762, 5.302) (9.2163, 5.2783) (9.1593, 5.2474) (9.1053, 5.21) (9.054, 5.1657) (9.0232, 5.1319) (9.0075, 5.1146) knots 0 0 0 0 0.128515 0.252949 0.374755 0.49594 0.617181 0.740909 0.867811 1 1 1 1
  line L46 (9.0075, 5.1146) -> (8.9054, 5.1919)
  spline S20 degree 3 poles (8.9054, 5.1919) (8.9136, 5.2025) (8.93, 5.2237) (8.9565, 5.2535) (8.9845, 5.2816) (9.0141, 5.3076) (9.045, 5.3322) (9.0777, 5.3546) (9.1118, 5.3751) (9.1472, 5.3939) (9.1839, 5.4106) (9.2218, 5.4249) (9.2607, 5.4372) (9.3007, 5.4473) (9.3418, 5.4552) (9.3839, 5.4605) (9.4271, 5.4641) (9.4563, 5.4644) (9.471, 5.4646) knots 0 0 0 0 0.061674 0.123053 0.183475 0.243727 0.304279 0.364863 0.425946 0.487391 0.54922 0.611144 0.673529 0.736961 0.800785 0.866013 0.932101 1 1 1 1
  spline S21 degree 3 poles (9.471, 5.4646) (9.485, 5.4645) (9.5126, 5.4643) (9.5535, 5.4612) (9.5932, 5.4569) (9.6318, 5.4505) (9.6693, 5.443) (9.7056, 5.4329) (9.7408, 5.4215) (9.775, 5.4082) (9.8081, 5.3931) (9.84, 5.3761) (9.8706, 5.3573) (9.9004, 5.3371) (9.9289, 5.3148) (9.9562, 5.2908) (9.9827, 5.2651) (9.999, 5.2466) (10.0072, 5.2373) knots 0 0 0 0 0.069663 0.13775 0.203917 0.26878 0.332414 0.394754 0.45618 0.516996 0.577396 0.637198 0.696999 0.756756 0.816554 0.876948 0.938132 1 1 1 1
  spline S22 degree 3 poles (10.0072, 5.2373) (10.0204, 5.2211) (10.0465, 5.1889) (10.08, 5.1368) (10.1087, 5.0824) (10.1318, 5.0254) (10.15, 4.966) (10.1625, 4.9041) (10.1707, 4.8397) (10.1716, 4.796) (10.1721, 4.7737) knots 0 0 0 0 0.124329 0.247156 0.36878 0.490734 0.613614 0.738958 0.867311 1 1 1 1
  line L47 (7.0994, 4.1813) -> (7.3122, 4.1813)
  line L48 (7.4998, 5.2813) -> (7.0994, 4.1813)
  line L49 (6.9998, 5.2813) -> (7.4998, 5.2813)
  line L50 (6.5994, 4.1813) -> (6.9998, 5.2813)
  line L51 (6.3866, 4.1813) -> (6.5994, 4.1813)
  line L52 (6.7869, 5.2813) -> (6.3866, 4.1813)
  line L53 (6.5869, 5.2813) -> (6.7869, 5.2813)
  line L54 (6.6597, 5.4813) -> (6.5869, 5.2813)
  line L55 (7.7854, 5.4813) -> (6.6597, 5.4813)
  line L56 (7.3122, 4.1813) -> (7.7854, 5.4813)
  line L57 (12.4754, 5.4313) -> (12.4921, 5.4313)
  line L58 (12.4921, 5.4313) -> (13.0421, 4.1313)
  line L59 (13.0421, 4.1313) -> (12.9171, 4.1313)
  line L60 (12.9171, 4.1313) -> (12.4837, 5.1557)
  line L61 (12.4837, 5.1557) -> (12.0504, 4.1313)
  line L62 (12.0504, 4.1313) -> (11.9254, 4.1313)
  line L63 (11.9254, 4.1313) -> (12.4754, 5.4313)
  spline S23 degree 3 poles (13.2854, 4.7818) (13.2856, 4.8017) (13.2861, 4.8404) (13.2886, 4.8971) (13.2934, 4.9505) (13.2994, 5.001) (13.3077, 5.0482) (13.318, 5.0923) (13.3294, 5.1335) (13.3434, 5.1715) (13.3588, 5.2067) (13.3755, 5.2397) (13.3935, 5.2706) (13.413, 5.2992) (13.4338, 5.3257) (13.4564, 5.3496) (13.48, 5.3716) (13.5051, 5.3912) (13.5312, 5.4083) (13.5579, 5.4236) (13.5857, 5.4359) (13.6139, 5.4465) (13.6429, 5.4546) (13.6727, 5.4602) (13.7032, 5.4641) (13.7238, 5.4644) (13.7341, 5.4646) knots 0 0 0 0 0.065063 0.126773 0.185516 0.240765 0.29298 0.34225 0.388919 0.432776 0.474628 0.514775 0.553606 0.591426 0.628028 0.663804 0.698984 0.733591 0.767628 0.801208 0.834264 0.866981 0.89972 0.932702 0.966176 1 1 1 1
  spline S24 degree 3 poles (13.7341, 5.4646) (13.7443, 5.4644) (13.7646, 5.4641) (13.7945, 5.4606) (13.8236, 5.4549) (13.8519, 5.4469) (13.8797, 5.4372) (13.9065, 5.4245) (13.9326, 5.4099) (13.9579, 5.3932) (13.9821, 5.3742) (14.0051, 5.3531) (14.0266, 5.3295) (14.0465, 5.3037) (14.0654, 5.2759) (14.0828, 5.2459) (14.0989, 5.2136) (14.1137, 5.1789) (14.1267, 5.1414) (14.1382, 5.1005) (14.1473, 5.0558) (14.1551, 5.0079) (14.1614, 4.9564) (14.1657, 4.9013) (14.1684, 4.8427) (14.1686, 4.8024) (14.1687, 4.7818) knots 0 0 0 0 0.033787 0.066622 0.099285 0.131361 0.163585 0.196104 0.228902 0.262158 0.295991 0.330218 0.36506 0.400951 0.43762 0.475708 0.515381 0.556414 0.599765 0.646424 0.696431 0.749782 0.806573 0.867436 0.931887 1 1 1 1
  spline S25 degree 3 poles (14.1687, 4.7818) (14.1686, 4.761) (14.1684, 4.7205) (14.1657, 4.6615) (14.1614, 4.6062) (14.1554, 4.5545) (14.1481, 4.5064) (14.1383, 4.4622) (14.1273, 4.4214) (14.1144, 4.3841) (14.1, 4.3497) (14.0842, 4.3176) (14.0665, 4.2879) (14.048, 4.26) (14.0277, 4.2344) (14.0065, 4.2107) (13.9833, 4.1896) (13.959, 4.1703) (13.9333, 4.1534) (13.9071, 4.1386) (13.8801, 4.1259) (13.8522, 4.1159) (13.8237, 4.1076) (13.7945, 4.102) (13.7646, 4.0984) (13.7443, 4.0981) (13.7341, 4.0979) knots 0 0 0 0 0.068595 0.133246 0.194313 0.251279 0.304513 0.354235 0.400481 0.443411 0.484015 0.523252 0.561042 0.5979 0.633518 0.668314 0.702496 0.736685 0.770293 0.803437 0.835913 0.86846 0.900847 0.933467 0.966258 1 1 1 1
  spline S26 degree 3 poles (13.7341, 4.0979) (13.7238, 4.0981) (13.7032, 4.0985) (13.6728, 4.1019) (13.6431, 4.1077) (13.6142, 4.1158) (13.586, 4.1259) (13.5585, 4.1386) (13.5317, 4.1533) (13.5059, 4.1706) (13.481, 4.19) (13.4574, 4.2118) (13.4352, 4.2359) (13.4142, 4.2621) (13.3948, 4.2908) (13.3764, 4.3215) (13.3599, 4.3548) (13.3441, 4.3902) (13.3304, 4.4286) (13.318, 4.4697) (13.308, 4.5141) (13.2997, 4.5616) (13.2933, 4.6122) (13.2886, 4.666) (13.2861, 4.7229) (13.2856, 4.7618) (13.2854, 4.7818) knots 0 0 0 0 0.033788 0.067194 0.099862 0.132567 0.165151 0.197913 0.231319 0.265083 0.299255 0.334399 0.369943 0.406284 0.444064 0.482998 0.523354 0.565537 0.609613 0.656391 0.705885 0.758325 0.813832 0.872795 0.934722 1 1 1 1
  line L64 (19.4354, 4.7813) -> (19.3021, 4.1313)
  line L65 (19.3021, 4.1313) -> (18.7687, 4.1313)
  line L66 (18.7687, 4.1313) -> (18.7687, 4.2646)
  line L67 (18.7687, 4.2646) -> (19.2109, 4.2646)
  line L68 (19.2109, 4.2646) -> (19.281, 4.6065)
  spline S27 degree 3 poles (19.281, 4.6065) (19.2672, 4.6027) (19.2405, 4.5954) (19.2012, 4.5872) (19.1638, 4.5823) (19.1396, 4.5816) (19.1278, 4.5813) knots 0 0 0 0 0.275068 0.532901 0.773973 1 1 1 1
  spline S28 degree 3 poles (19.1278, 4.5813) (19.1133, 4.5816) (19.0848, 4.5822) (19.043, 4.5881) (19.0032, 4.5975) (18.9653, 4.6105) (18.9293, 4.6272) (18.8956, 4.648) (18.8636, 4.6724) (18.8339, 4.7004) (18.8069, 4.7312) (18.7832, 4.7643) (18.7631, 4.7994) (18.7469, 4.8368) (18.734, 4.8762) (18.7254, 4.9179) (18.7197, 4.9615) (18.7191, 4.9913) (18.7187, 5.0065) knots 0 0 0 0 0.065808 0.129394 0.190894 0.251281 0.310815 0.370371 0.430768 0.492881 0.555104 0.616067 0.677256 0.73826 0.800762 0.864778 0.931045 1 1 1 1
  spline S29 degree 3 poles (18.7187, 5.0065) (18.719, 5.0171) (18.7195, 5.0382) (18.722, 5.0694) (18.7268, 5.1) (18.7332, 5.1299) (18.7416, 5.1592) (18.7517, 5.1878) (18.7641, 5.2155) (18.7777, 5.2428) (18.7931, 5.2688) (18.8101, 5.2932) (18.828, 5.3163) (18.8474, 5.3378) (18.8682, 5.3576) (18.8904, 5.3757) (18.9137, 5.3926) (18.9384, 5.4075) (18.9641, 5.4213) (18.9911, 5.4325) (19.0187, 5.4426) (19.0475, 5.4506) (19.0772, 5.4569) (19.108, 5.4612) (19.1398, 5.4643) (19.1613, 5.4645) (19.1721, 5.4646) knots 0 0 0 0 0.044014 0.087434 0.130118 0.172554 0.214555 0.256298 0.298438 0.340849 0.382715 0.423924 0.464246 0.504074 0.543862 0.583567 0.623094 0.663229 0.703551 0.743938 0.784541 0.82575 0.867757 0.910745 0.954914 1 1 1 1
  spline S30 degree 3 poles (19.1721, 5.4646) (19.1851, 5.4643) (19.2106, 5.4638) (19.2479, 5.4586) (19.2838, 5.451) (19.318, 5.4396) (19.3509, 5.4254) (19.3818, 5.4073) (19.4118, 5.3869) (19.4395, 5.3628) (19.4651, 5.3365) (19.4881, 5.3079) (19.5086, 5.2775) (19.5262, 5.2453) (19.5413, 5.2111) (19.5531, 5.1751) (19.5626, 5.1372) (19.5667, 5.1112) (19.5687, 5.0979) knots 0 0 0 0 0.065421 0.128708 0.190236 0.250724 0.310637 0.370766 0.431615 0.493523 0.555883 0.617342 0.678668 0.740711 0.802985 0.866803 0.932347 1 1 1 1
  line L69 (19.5687, 5.0979) -> (19.4521, 5.0979)
  spline S31 degree 3 poles (19.4521, 5.0979) (19.4492, 5.1103) (19.4437, 5.1342) (19.4316, 5.1676) (19.4168, 5.1975) (19.3991, 5.2241) (19.3781, 5.2472) (19.3542, 5.2679) (19.3273, 5.2865) (19.2974, 5.3021) (19.2659, 5.3153) (19.233, 5.3241) (19.1994, 5.3303) (19.1767, 5.331) (19.1653, 5.3313) knots 0 0 0 0 0.094687 0.181994 0.264377 0.34218 0.418618 0.496509 0.577369 0.661511 0.746733 0.831258 0.915206 1 1 1 1
  spline S32 degree 3 poles (19.1653, 5.3313) (19.1542, 5.331) (19.1323, 5.3304) (19.1001, 5.3257) (19.0689, 5.3186) (19.0392, 5.308) (19.0104, 5.295) (18.9832, 5.2784) (18.9569, 5.2593) (18.9322, 5.2374) (18.9096, 5.2133) (18.8897, 5.1875) (18.873, 5.1599) (18.859, 5.1312) (18.8484, 5.1008) (18.8408, 5.0691) (18.8363, 5.0358) (18.8357, 5.0131) (18.8354, 5.0016) knots 0 0 0 0 0.064207 0.126425 0.18768 0.248216 0.308305 0.369661 0.431699 0.495947 0.559758 0.622295 0.683911 0.745092 0.80674 0.869087 0.93329 1 1 1 1
  spline S33 degree 3 poles (18.8354, 5.0016) (18.8356, 4.9912) (18.8361, 4.9707) (18.84, 4.9409) (18.8468, 4.9126) (18.8563, 4.8858) (18.8683, 4.8605) (18.8829, 4.8366) (18.9005, 4.8144) (18.9206, 4.7939) (18.9426, 4.775) (18.9669, 4.7589) (18.993, 4.7454) (19.0206, 4.7337) (19.0503, 4.7253) (19.0815, 4.719) (19.1147, 4.7154) (19.1373, 4.7149) (19.1489, 4.7146) knots 0 0 0 0 0.065351 0.127916 0.18836 0.247216 0.30563 0.36377 0.422661 0.482687 0.5433 0.604118 0.664965 0.727413 0.791468 0.858055 0.927037 1 1 1 1
  spline S34 degree 3 poles (19.1489, 4.7146) (19.159, 4.7148) (19.1798, 4.7153) (19.2117, 4.7185) (19.2453, 4.7238) (19.2803, 4.7311) (19.3169, 4.7406) (19.3551, 4.752) (19.3948, 4.7657) (19.4216, 4.776) (19.4354, 4.7813) knots 0 0 0 0 0.102203 0.211023 0.3251 0.446502 0.573788 0.708901 0.850358 1 1 1 1
  line L70 (0, 80) -> (0, 0) projected
  line L71 (0, 40) -> (8.6448, 40)
  line L72 (1.9345, 80.1187) -> (2.4471, 80.1187)
  line L73 (2.4471, 80.1187) -> (2.5388, 78.6847)
  arc A17 (2.5388, 78.6847) -> (6.7302, 78.6847) centre (4.6345, 78.8187) ccw
  line L74 (6.7302, 78.6847) -> (6.8219, 80.1187)
  line L75 (6.8219, 80.1187) -> (11.1103, 80.1187)
  arc A18 (11.181, 80.0894) -> (11.1103, 80.1187) centre (11.1103, 80.0187) ccw
  line L76 (11.181, 80.0894) -> (11.5052, 79.7652)
  arc A19 (11.5052, 79.7652) -> (11.8588, 79.6187) centre (11.8588, 80.1187) ccw
  line L77 (11.8588, 79.6187) -> (21.5345, 79.6187)
  arc A20 (21.4407, 79.5534) -> (21.5345, 79.6187) centre (21.5345, 79.5187) ccw
  line L78 (21.4407, 79.5534) -> (21.4407, 70.4583)
  arc A21 (21.4519, 70.2687) -> (21.4407, 70.4583) centre (21.5345, 70.3687) ccw
  line L79 (21.4519, 70.2687) -> (18.6088, 70.2687)
  arc A22 (18.6088, 70.2687) -> (18.2552, 70.1223) centre (18.6088, 69.7687) ccw
  line L80 (18.2552, 70.1223) -> (17.931, 69.798)
  arc A23 (17.8603, 69.7687) -> (17.931, 69.798) centre (17.8603, 69.8687) ccw
  line L81 (17.8603, 69.7687) -> (15.1088, 69.7687)
  arc A24 (15.0381, 69.798) -> (15.1088, 69.7687) centre (15.1088, 69.8687) ccw
  line L82 (15.0381, 69.798) -> (14.7138, 70.1223)
  arc A25 (14.7138, 70.1223) -> (14.3603, 70.2687) centre (14.3603, 69.7687) ccw
  line L83 (14.3603, 70.2687) -> (9.1088, 70.2687)
  arc A26 (9.1088, 70.2687) -> (8.7552, 70.1223) centre (9.1088, 69.7687) ccw
  line L84 (8.7552, 70.1223) -> (8.431, 69.798)
  arc A27 (8.3603, 69.7687) -> (8.431, 69.798) centre (8.3603, 69.8687) ccw
  line L85 (8.3603, 69.7687) -> (5.6088, 69.7687)
  arc A28 (5.5381, 69.798) -> (5.6088, 69.7687) centre (5.6088, 69.8687) ccw
  line L86 (5.5381, 69.798) -> (5.2138, 70.1223)
  arc A29 (5.2138, 70.1223) -> (4.8603, 70.2687) centre (4.8603, 69.7687) ccw
  line L87 (4.8603, 70.2687) -> (1.9345, 70.2687)
  arc A30 (2.0046, 70.4401) -> (1.9345, 70.2687) centre (1.9345, 70.3687) ccw
  line L88 (2.0046, 70.4401) -> (2.0046, 79.9474)
  arc A31 (1.9345, 80.1187) -> (2.0046, 79.9474) centre (1.9345, 80.0187) ccw
  circle A32 centre (7.7854, 72.3187) radius 1.25
  circle A33 centre (17.2854, 72.3187) radius 1.25
  line L89 (18.4587, 74.5687) -> (17.8421, 75.8687)
  line L90 (17.8421, 75.8687) -> (17.8254, 75.8687)
  line L91 (17.8254, 75.8687) -> (17.2254, 74.5687)
  line L92 (17.2254, 74.5687) -> (17.3522, 74.5687)
  line L93 (17.3522, 74.5687) -> (17.5444, 74.9854)
  line L94 (17.5444, 74.9854) -> (18.1337, 74.9854)
  line L95 (18.1337, 74.9854) -> (18.3314, 74.5687)
  line L96 (18.3314, 74.5687) -> (18.4587, 74.5687)
  spline S35 degree 3 poles (15.6387, 75.5052) (15.639, 75.5141) (15.6394, 75.5315) (15.6435, 75.5572) (15.6497, 75.5819) (15.6586, 75.6058) (15.6704, 75.6286) (15.6847, 75.6504) (15.7012, 75.6715) (15.7202, 75.6912) (15.7412, 75.7093) (15.7633, 75.7253) (15.7867, 75.7387) (15.8113, 75.7497) (15.8371, 75.7583) (15.8639, 75.7642) (15.8919, 75.768) (15.911, 75.7685) (15.9208, 75.7687) knots 0 0 0 0 0.061965 0.122122 0.180988 0.239933 0.299906 0.359989 0.421776 0.486576 0.551535 0.615018 0.677259 0.73973 0.80305 0.866495 0.931973 1 1 1 1
  spline S36 degree 3 poles (15.9208, 75.7687) (15.9309, 75.7685) (15.9509, 75.7679) (15.9802, 75.7643) (16.0082, 75.758) (16.0349, 75.7494) (16.0603, 75.7385) (16.0844, 75.7248) (16.1071, 75.7086) (16.1284, 75.6901) (16.148, 75.6696) (16.1653, 75.6467) (16.1803, 75.6219) (16.1935, 75.5952) (16.2042, 75.5664) (16.2123, 75.5356) (16.2188, 75.5029) (16.221, 75.4803) (16.2221, 75.4687) knots 0 0 0 0 0.064439 0.126547 0.186887 0.245878 0.304041 0.362191 0.420976 0.48066 0.5406 0.600689 0.661936 0.724443 0.789038 0.856314 0.926352 1 1 1 1
  line L97 (16.2221, 75.4687) -> (16.3387, 75.4687)
  spline S37 degree 3 poles (16.3387, 75.4687) (16.338, 75.4842) (16.3365, 75.5146) (16.3295, 75.5589) (16.3195, 75.6013) (16.3053, 75.6414) (16.2878, 75.6795) (16.2667, 75.7155) (16.2417, 75.7493) (16.2134, 75.7806) (16.1827, 75.8092) (16.1495, 75.834) (16.1147, 75.8549) (16.0782, 75.8724) (16.0398, 75.8855) (15.9997, 75.8953) (15.9578, 75.9011) (15.9293, 75.9017) (15.9148, 75.9021) knots 0 0 0 0 0.068791 0.135103 0.198979 0.261904 0.323495 0.385195 0.446969 0.509765 0.572251 0.633405 0.693251 0.752583 0.812579 0.873275 0.93555 1 1 1 1
  spline S38 degree 3 poles (15.9148, 75.9021) (15.9005, 75.9017) (15.8725, 75.9011) (15.8316, 75.8954) (15.7927, 75.8866) (15.7558, 75.8743) (15.7213, 75.8576) (15.6888, 75.8376) (15.658, 75.8145) (15.6303, 75.7873) (15.6049, 75.7583) (15.5829, 75.7273) (15.5641, 75.6952) (15.5485, 75.6619) (15.5369, 75.6271) (15.5282, 75.5911) (15.5232, 75.5538) (15.5224, 75.5285) (15.5221, 75.5156) knots 0 0 0 0 0.069475 0.136517 0.200789 0.26383 0.325735 0.387291 0.449509 0.512968 0.576275 0.63758 0.697903 0.757172 0.816599 0.876653 0.93729 1 1 1 1
  spline S39 degree 3 poles (15.5221, 75.5156) (15.5227, 75.4975) (15.5239, 75.4616) (15.5346, 75.4089) (15.5513, 75.3578) (15.5713, 75.3166) (15.5915, 75.2835) (15.6098, 75.2562) (15.6311, 75.2268) (15.6559, 75.1954) (15.6836, 75.1618) (15.7144, 75.126) (15.7486, 75.0883) (15.7726, 75.0625) (15.7851, 75.0492) knots 0 0 0 0 0.098702 0.195672 0.292422 0.391343 0.444462 0.504229 0.570352 0.642546 0.722288 0.807921 0.90047 1 1 1 1
  line L98 (15.7851, 75.0492) -> (16.1103, 74.7021)
  line L99 (16.1103, 74.7021) -> (15.5054, 74.7021)
  line L100 (15.5054, 74.7021) -> (15.5054, 74.5687)
  line L101 (15.5054, 74.5687) -> (16.3887, 74.5687)
  line L102 (16.3887, 74.5687) -> (15.8846, 75.1068)
  spline S40 degree 3 poles (15.8846, 75.1068) (15.8723, 75.1196) (15.8487, 75.1442) (15.8154, 75.1801) (15.7854, 75.2134) (15.7587, 75.2441) (15.7357, 75.2726) (15.7153, 75.2979) (15.699, 75.3212) (15.6813, 75.3482) (15.6641, 75.3812) (15.6493, 75.4215) (15.6404, 75.463) (15.6393, 75.4911) (15.6387, 75.5052) knots 0 0 0 0 0.110803 0.212829 0.306101 0.390647 0.466924 0.534481 0.593587 0.644557 0.7362 0.825024 0.911986 1 1 1 1
  line L103 (15.1287, 75.2187) -> (14.9954, 75.8687)
  line L104 (14.9954, 75.8687) -> (14.4621, 75.8687)
  line L105 (14.4621, 75.8687) -> (14.4621, 75.7354)
  line L106 (14.4621, 75.7354) -> (14.9042, 75.7354)
  line L107 (14.9042, 75.7354) -> (14.9743, 75.3935)
  spline S41 degree 3 poles (14.9743, 75.3935) (14.9605, 75.3973) (14.9339, 75.4046) (14.8945, 75.4128) (14.8572, 75.4177) (14.8329, 75.4184) (14.8212, 75.4187) knots 0 0 0 0 0.275068 0.532901 0.773973 1 1 1 1
  spline S42 degree 3 poles (14.8212, 75.4187) (14.8067, 75.4184) (14.7781, 75.4178) (14.7364, 75.4119) (14.6965, 75.4025) (14.6586, 75.3895) (14.6226, 75.3728) (14.5889, 75.352) (14.5569, 75.3276) (14.5272, 75.2996) (14.5003, 75.2688) (14.4766, 75.2357) (14.4565, 75.2006) (14.4403, 75.1632) (14.4274, 75.1238) (14.4188, 75.0821) (14.413, 75.0385) (14.4124, 75.0087) (14.4121, 74.9935) knots 0 0 0 0 0.065808 0.129394 0.190894 0.251281 0.310815 0.370371 0.430768 0.492881 0.555104 0.616067 0.677256 0.73826 0.800762 0.864778 0.931045 1 1 1 1
  spline S43 degree 3 poles (14.4121, 74.9935) (14.4123, 74.9829) (14.4128, 74.9618) (14.4153, 74.9306) (14.4201, 74.9) (14.4266, 74.8701) (14.4349, 74.8408) (14.4451, 74.8122) (14.4575, 74.7845) (14.4711, 74.7572) (14.4864, 74.7312) (14.5034, 74.7068) (14.5214, 74.6837) (14.5407, 74.6622) (14.5616, 74.6424) (14.5837, 74.6243) (14.607, 74.6074) (14.6318, 74.5925) (14.6574, 74.5787) (14.6844, 74.5675) (14.7121, 74.5574) (14.7408, 74.5494) (14.7706, 74.5431) (14.8014, 74.5388) (14.8331, 74.5357) (14.8546, 74.5355) (14.8654, 74.5354) knots 0 0 0 0 0.044014 0.087434 0.130118 0.172554 0.214555 0.256298 0.298438 0.340849 0.382715 0.423924 0.464246 0.504074 0.543862 0.583567 0.623094 0.663229 0.703551 0.743938 0.784541 0.82575 0.867757 0.910745 0.954914 1 1 1 1
  spline S44 degree 3 poles (14.8654, 74.5354) (14.8784, 74.5357) (14.9039, 74.5362) (14.9412, 74.5414) (14.9771, 74.549) (15.0114, 74.5604) (15.0442, 74.5746) (15.0752, 74.5927) (15.1051, 74.6131) (15.1328, 74.6372) (15.1585, 74.6635) (15.1815, 74.6921) (15.2019, 74.7225) (15.2196, 74.7547) (15.2346, 74.7889) (15.2464, 74.8249) (15.256, 74.8628) (15.26, 74.8888) (15.2621, 74.9021) knots 0 0 0 0 0.065421 0.128708 0.190236 0.250724 0.310637 0.370766 0.431615 0.493523 0.555883 0.617342 0.678668 0.740711 0.802985 0.866803 0.932347 1 1 1 1
  line L108 (15.2621, 74.9021) -> (15.1454, 74.9021)
  spline S45 degree 3 poles (15.1454, 74.9021) (15.1425, 74.8897) (15.137, 74.8658) (15.1249, 74.8324) (15.1101, 74.8025) (15.0925, 74.7759) (15.0715, 74.7528) (15.0475, 74.7321) (15.0206, 74.7135) (14.9908, 74.6979) (14.9593, 74.6847) (14.9263, 74.6759) (14.8928, 74.6697) (14.8701, 74.669) (14.8587, 74.6687) knots 0 0 0 0 0.094687 0.181994 0.264377 0.34218 0.418618 0.496509 0.577369 0.661511 0.746733 0.831258 0.915206 1 1 1 1
  spline S46 degree 3 poles (14.8587, 74.6687) (14.8475, 74.669) (14.8256, 74.6696) (14.7934, 74.6743) (14.7623, 74.6814) (14.7326, 74.692) (14.7037, 74.705) (14.6766, 74.7216) (14.6502, 74.7407) (14.6256, 74.7626) (14.603, 74.7867) (14.583, 74.8125) (14.5664, 74.8401) (14.5523, 74.8688) (14.5417, 74.8992) (14.5341, 74.9309) (14.5297, 74.9642) (14.529, 74.9869) (14.5287, 74.9984) knots 0 0 0 0 0.064207 0.126425 0.18768 0.248216 0.308305 0.369661 0.431699 0.495947 0.559758 0.622295 0.683911 0.745092 0.80674 0.869087 0.93329 1 1 1 1
  spline S47 degree 3 poles (14.5287, 74.9984) (14.529, 75.0088) (14.5295, 75.0293) (14.5334, 75.0591) (14.5402, 75.0874) (14.5496, 75.1142) (14.5616, 75.1395) (14.5763, 75.1634) (14.5938, 75.1856) (14.6139, 75.2061) (14.6359, 75.225) (14.6602, 75.2411) (14.6863, 75.2546) (14.7139, 75.2663) (14.7436, 75.2747) (14.7749, 75.281) (14.808, 75.2846) (14.8306, 75.2851) (14.8423, 75.2854) knots 0 0 0 0 0.065351 0.127916 0.18836 0.247216 0.30563 0.36377 0.422661 0.482687 0.5433 0.604118 0.664965 0.727413 0.791468 0.858055 0.927037 1 1 1 1